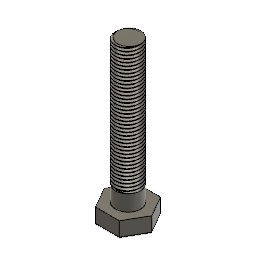
13part (Autodesk Fusion 360 design; units mm, degrees)
Autodesk Fusion 360 part; units mm, degrees
sketch "Sketch1" plane through (0, 0, 0) normal (0, 1, 0) x (1, 0, 0)
  circle A0 centre (0, 0) radius 4
  line L0 (-3.7528, 6.5) -> (-7.5056, 0)
  line L1 (-7.5056, 0) -> (-3.7528, -6.5)
  line L2 (-3.7528, -6.5) -> (3.7528, -6.5)
  line L3 (3.7528, -6.5) -> (7.5056, 0)
  line L4 (7.5056, 0) -> (3.7528, 6.5)
  line L5 (3.7528, 6.5) -> (-3.7528, 6.5)
  dimension "d1" = 8
  dimension "d2" = 6.5
  constraint coincident A0.centre origin
  constraint horizontal L5
  measures "d1" diameter of A0
  measures "d2" distance of A0.centre L5
extrude "Extrude1" add sketch "Sketch1" along normal blind 50 contours A0
extrude "Extrude2" add sketch "Sketch1" along normal blind 5
fillet "Fillet1" radius 0.5 1 faces at (-2.5019, 0, 0)
thread "Thread1" "ISO Metric profile 8.0 M8x1 6g" major diameter 7.884 minor diameter 6.7435 pitch 1 angle 60 modelled right hand crest width 0.125 on face at (3.9801, 20, 0.3983) from (0, 10, 0) to (0, 50, 0) crest through (3.942, 4.9375, 0)
